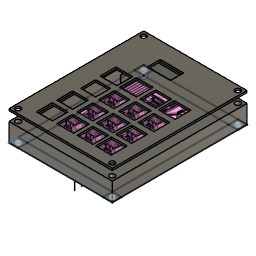
cALCULATOR TOP + BOTTOM v2 (Autodesk Fusion 360 design; units mm, degrees)
Autodesk Fusion 360 part; units mm, degrees
sketch "Sketch1" plane through (0, 0, 0) normal (0, 0, 1) x (1, 0, 0)
  line L0 (0, 0) -> (92, 0)
  line L1 (92, 0) -> (92, -126)
  line L2 (92, -126) -> (0, -126)
  line L3 (0, -126) -> (0, 0)
  line L4 (92, -126) -> (102, -126)
  line L5 (102, -126) -> (102, -136)
  line L6 (102, -136) -> (92, -136)
  line L7 (92, -136) -> (92, -126)
  line L8 (0, -126) -> (-10, -126)
  line L9 (-10, -126) -> (-10, -136)
  line L10 (-10, -136) -> (0, -136)
  line L11 (0, -136) -> (0, -126)
  line L12 (0, 0) -> (-10, 0)
  line L13 (-10, 0) -> (-10, 10)
  line L14 (-10, 10) -> (0, 10)
  line L15 (0, 10) -> (0, 0)
  line L16 (92, 0) -> (102, 0)
  line L17 (102, 0) -> (102, 10)
  line L18 (102, 10) -> (92, 10)
  line L19 (92, 10) -> (92, 0)
  line L20 (102, -136) -> (-10, -136)
  line L21 (-10, -136) -> (-10, 10)
  line L22 (-10, 10) -> (102, 10)
  line L23 (102, 10) -> (102, -136)
  circle A0 centre (-5, 5) radius 2.85
  circle A1 centre (97, 5) radius 2.85
  circle A2 centre (97, -131) radius 2.85
  circle A3 centre (-5, -131) radius 2.85
  dimension "d1" = 92
  dimension "d2" = 126
  dimension "d3" = 10
  dimension "d4" = 10
  dimension "d5" = 10
  dimension "d6" = 10
  dimension "d7" = 10
  dimension "d8" = 10
  dimension "d9" = 10
  dimension "d10" = 5.7
  dimension "d11" = 5.7
  dimension "d12" = 5.7
  dimension "d13" = 5.7
  constraint horizontal L0
  constraint vertical L1
  constraint horizontal L2
  constraint vertical L3
  constraint coincident L0.start L3.end
  constraint horizontal L4
  constraint vertical L5
  constraint horizontal L6
  constraint vertical L7
  constraint horizontal L8
  constraint vertical L9
  constraint horizontal L10
  constraint vertical L11
  constraint horizontal L12
  constraint vertical L13
  constraint horizontal L14
  constraint vertical L15
  constraint horizontal L16
  constraint vertical L17
  constraint horizontal L18
  constraint vertical L19
  constraint horizontal L20
  constraint vertical L21
  constraint horizontal L22
  constraint vertical L23
  measures "d1" distance of L0.start L0.end
  measures "d2" distance of L0.start L2.end
  measures "d3" distance of L1.end L4.end
  measures "d4" distance of L1.end L6.end
  measures "d5" distance of L2.end L10.end
  measures "d6" distance of L0.start L12.end
  measures "d7" distance of L0.start L14.end
  measures "d8" distance of L0.end L16.end
  measures "d9" distance of L0.end L18.end
  measures "d10" diameter of A0
  measures "d11" diameter of A1
  measures "d12" diameter of A2
  measures "d13" diameter of A3
extrude "Extrude4" add sketch "Sketch1" along normal blind 20 contours L0 L15 L19 L22 | L3 L8 L12 L21 | L12 L13 L14 L15 L21 L22 | L1 L4 L16 L23 | L16 L17 L18 L19 L22 L23 | L8 L9 L10 L11 L20 L21 | L2 L7 L11 L20 | L4 L5 L6 L7 L20 L23 makes body 1
extrude "Extrude5" add sketch "Sketch1" along normal blind 1 contours L0 L1 L2 L3 bodies 1
extrude "Extrude6" add sketch "Sketch1" along normal blind 15 contours A0 | A1 | A2 | A3 bodies 1
other "Base Mesh Feature2"
sketch "Sketch2" plane through (0, 0, 20) normal (0, 0, 1) x (-1, 0, 0)
  circle A0 centre (-97, 131) radius 2.85
  circle A1 centre (5, 131) radius 2.85
  line L0 (-92, 126) -> (0, 126)
  line L1 (0, 126) -> (0, 0)
  line L2 (0, 0) -> (-92, 0)
  line L3 (-92, 0) -> (-92, 126)
  circle A2 centre (5, -5) radius 2.85
  circle A3 centre (-97, -5) radius 2.85
  line L4 (-102, -10) -> (10, -10)
  line L5 (10, -10) -> (10, 136)
  line L6 (10, 136) -> (-102, 136)
  line L7 (-102, 136) -> (-102, -10)
  line L8 (10, -10) -> (-102, -10)
  line L9 (-102, -10) -> (-102, 136)
  line L10 (-102, 136) -> (10, 136)
  line L11 (10, 136) -> (10, -10)
  line L12 (-26, 8) -> (-51, 8)
  line L13 (-51, 8) -> (-51, 22)
  line L14 (-51, 22) -> (-26, 22)
  line L15 (-26, 22) -> (-26, 8)
  line L16 (-9, 39) -> (-27, 39)
  line L17 (-27, 39) -> (-27, 56)
  line L18 (-27, 56) -> (-9, 56)
  line L19 (-9, 56) -> (-9, 39)
  line L20 (-30, 56) -> (-48, 56)
  line L21 (-48, 56) -> (-48, 38)
  line L22 (-48, 38) -> (-30, 38)
  line L23 (-30, 38) -> (-30, 56)
  line L24 (-52, 39) -> (-69, 39)
  line L25 (-69, 39) -> (-69, 56)
  line L26 (-69, 56) -> (-52, 56)
  line L27 (-52, 56) -> (-52, 39)
  line L28 (-72, 56) -> (-90, 56)
  line L29 (-90, 56) -> (-90, 39)
  line L30 (-90, 39) -> (-72, 39)
  line L31 (-72, 39) -> (-72, 56)
  line L32 (-73, 62) -> (-90, 62)
  line L33 (-90, 62) -> (-90, 79)
  line L34 (-90, 79) -> (-73, 79)
  line L35 (-73, 79) -> (-73, 62)
  line L36 (-69, 79) -> (-52, 79)
  line L37 (-52, 79) -> (-52, 61)
  line L38 (-52, 61) -> (-69, 61)
  line L39 (-69, 61) -> (-69, 79)
  line L40 (-47, 62) -> (-30.3345, 62)
  line L41 (-30.3345, 62) -> (-30.3345, 79)
  line L42 (-30.3345, 79) -> (-47, 79)
  line L43 (-47, 79) -> (-47, 62)
  line L44 (-26, 78) -> (-10, 78)
  line L45 (-10, 78) -> (-10, 62)
  line L46 (-10, 62) -> (-26, 62)
  line L47 (-26, 62) -> (-26, 78)
  line L48 (-8, 85) -> (-25, 85)
  line L49 (-25, 85) -> (-25, 102)
  line L50 (-25, 102) -> (-8, 102)
  line L51 (-8, 102) -> (-8, 85)
  line L52 (-30, 102) -> (-47, 102)
  line L53 (-47, 102) -> (-47, 85)
  line L54 (-47, 85) -> (-30, 85)
  line L55 (-30, 85) -> (-30, 102)
  line L56 (-51, 84) -> (-69, 84)
  line L57 (-69, 84) -> (-69, 102)
  line L58 (-69, 102) -> (-51, 102)
  line L59 (-51, 102) -> (-51, 84)
  line L60 (-72, 85) -> (-89, 85)
  line L61 (-89, 85) -> (-89, 102)
  line L62 (-89, 102) -> (-72, 102)
  line L63 (-72, 102) -> (-72, 85)
  line L64 (-72, 107) -> (-89, 107)
  line L65 (-89, 107) -> (-89, 124)
  line L66 (-89, 124) -> (-72, 124)
  line L67 (-72, 124) -> (-72, 107)
  line L68 (-69, 124) -> (-52, 124)
  line L69 (-52, 124) -> (-52, 107)
  line L70 (-52, 107) -> (-69, 107)
  line L71 (-69, 107) -> (-69, 124)
  line L72 (-48, 107) -> (-30, 107)
  line L73 (-30, 107) -> (-30, 124)
  line L74 (-30, 124) -> (-48, 124)
  line L75 (-48, 124) -> (-48, 107)
  line L76 (-25, 124) -> (-8, 124)
  line L77 (-8, 124) -> (-8, 107)
  line L78 (-8, 107) -> (-25, 107)
  line L79 (-25, 107) -> (-25, 124)
  constraint horizontal L8
  constraint vertical L9
  constraint horizontal L10
  constraint vertical L11
  constraint coincident L6.end L7.start
  constraint coincident L4.end L5.start
  constraint horizontal L12
  constraint vertical L13
  constraint horizontal L14
  constraint vertical L15
  constraint horizontal L16
  constraint vertical L17
  constraint horizontal L18
  constraint vertical L19
  constraint horizontal L20
  constraint vertical L21
  constraint horizontal L22
  constraint vertical L23
  constraint horizontal L24
  constraint vertical L25
  constraint horizontal L26
  constraint vertical L27
  constraint horizontal L28
  constraint vertical L29
  constraint horizontal L30
  constraint vertical L31
  constraint horizontal L32
  constraint vertical L33
  constraint horizontal L34
  constraint vertical L35
  constraint horizontal L36
  constraint vertical L37
  constraint horizontal L38
  constraint vertical L39
  constraint horizontal L40
  constraint vertical L41
  constraint horizontal L42
  constraint vertical L43
  constraint horizontal L44
  constraint vertical L45
  constraint horizontal L46
  constraint vertical L47
  constraint horizontal L48
  constraint vertical L49
  constraint horizontal L50
  constraint vertical L51
  constraint horizontal L52
  constraint vertical L53
  constraint horizontal L54
  constraint vertical L55
  constraint horizontal L56
  constraint vertical L57
  constraint horizontal L58
  constraint vertical L59
  constraint horizontal L60
  constraint vertical L61
  constraint horizontal L62
  constraint vertical L63
  constraint horizontal L64
  constraint vertical L65
  constraint horizontal L66
  constraint vertical L67
  constraint horizontal L68
  constraint vertical L69
  constraint horizontal L70
  constraint vertical L71
  constraint horizontal L72
  constraint vertical L73
  constraint horizontal L74
  constraint vertical L75
  constraint horizontal L76
  constraint vertical L77
  constraint horizontal L78
  constraint vertical L79
extrude "Extrude7" add sketch "Sketch2" along normal blind 2 separate body contours L0 L1 L2 L3 | L4 L5 L6 L7 L8 L9 L10 L11 makes body 2
move_body "Move1" bodies 2 to x (1, 0, 0) y (0, 1, 0) z (0, 0, 1) at (0, 0, 10)
sketch "Sketch3" plane through (0, 0, 20) normal (0, 0, 1) x (-1, 0, 0)
  circle A0 centre (-97, 131) radius 2.85
  circle A1 centre (5, 131) radius 2.85
  line L0 (-92, 126) -> (0, 126)
  line L1 (0, 126) -> (0, 0)
  line L2 (0, 0) -> (-92, 0)
  line L3 (-92, 0) -> (-92, 126)
  circle A2 centre (5, -5) radius 2.85
  circle A3 centre (-97, -5) radius 2.85
  line L4 (-102, -10) -> (10, -10)
  line L5 (10, -10) -> (10, 136)
  line L6 (10, 136) -> (-102, 136)
  line L7 (-102, 136) -> (-102, -10)
  line L8 (10, 10) -> (0, 10)
  line L9 (0, 10) -> (0, 25)
  line L10 (0, 25) -> (10, 25)
  line L11 (10, 25) -> (10, 10)
  line L12 (-62, 0) -> (-70, 0)
  line L13 (-70, 0) -> (-70, -10)
  line L14 (-70, -10) -> (-62, -10)
  line L15 (-62, -10) -> (-62, 0)
  constraint horizontal L8
  constraint vertical L9
  constraint horizontal L10
  constraint vertical L11
  constraint coincident L1 L9.end
  constraint coincident L5 L8.start
  constraint horizontal L12
  constraint vertical L13
  constraint horizontal L14
  constraint vertical L15
  constraint coincident L4 L13.end
  constraint coincident L2 L12.start
extrude "Extrude8" cut sketch "Sketch3" along normal blind 5 and the other way blind 5 from surface at -12 contours L1 L5 L8 L9 L10 L11 | L2 L4 L12 L13 L14 L15 bodies 1
